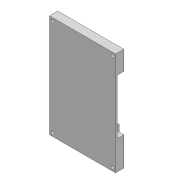
# Autodesk Inventor part: DE10-Nano
Saved by Autodesk Inventor 2018 (Build 220112000, 112)
## iProperties
Created: 2019-08-31
Part Number: DE10-Nano
Material: Generic
Document SubType Name: Modeling
Designer: Clevo
Density: 1 g/cm^3
Appearance: Default
Author: Clevo
Autodesk Inventor part; units mm, degrees
ref_plane "YZ Plane" through (0, 0, 0) normal (1, 0, 0) x (0, 1, 0)
ref_plane "XZ Plane" through (0, 0, 0) normal (0, 1, 0) x (-1, 0, 0)
ref_plane "XY Plane" through (0, 0, 0) normal (0, 0, 1) x (1, 0, 0)
sketch "Sketch1" plane through (0, 0, 0) normal (0, 1, 0) x (-1, 0, 0)
  line L0 (-34.295, -53.46) -> (34.295, -53.46)
  line L1 (34.295, -53.46) -> (34.295, 53.46)
  line L2 (34.295, 53.46) -> (-34.295, 53.46)
  line L3 (-34.295, 53.46) -> (-34.295, -53.46)
  line L4 (-34.295, -53.46) -> (34.295, 53.46) construction
  line L5 (34.295, -53.46) -> (-34.295, 53.46) construction
  point P0 (0, 0)
  dimension "d0" = 106.92
  dimension "d1" = 68.59
  constraints: 12 end point, 2 midpoint, 2 parallel, 1 horizontal, 1 perpendicular
  measures "d0" distance of L0.end L1.end
  measures "d1" distance of L1.end L2.end
extrude "Extrusion1" add sketch "Sketch1" along normal blind 1.6
sketch "Sketch2" plane through (0, 1.6, 0) normal (0, 1, 0) x (1, 0, 0)
  line L0 (-34.295, 53.46) -> (-34.295, -53.46) projected
  line L1 (34.295, -53.46) -> (34.295, 53.46) projected
  line L2 (-34.295, -53.46) -> (34.295, -53.46)
  line L3 (34.295, -53.46) -> (34.295, -33.46)
  line L4 (34.295, -33.46) -> (-34.295, -33.46)
  line L5 (-34.295, -33.46) -> (-34.295, -53.46)
  line L6 (34.295, 53.46) -> (-34.295, 53.46) projected
  line L7 (34.295, 53.46) -> (-34.295, 53.46)
  line L8 (-34.295, 53.46) -> (-34.295, 23.46)
  line L9 (-34.295, 23.46) -> (34.295, 23.46)
  line L10 (34.295, 23.46) -> (34.295, 53.46)
  point P0 (0, 0)
  dimension "d4" = 20
  dimension "d5" = 30
  constraints: 16 end point, 4 parallel, 2 horizontal, 2 perpendicular, 2 point on line
  measures "d4" distance between parallel lines of L2 L4
  measures "d5" distance between parallel lines of L6 L9
extrude "Extrusion2" add sketch "Sketch2" along normal blind 7 contours L6 L1 L9 L0 | L4 L1 L2 L0
sketch "Sketch3" plane through (0, 8.6, 0) normal (0, 1, 0) x (1, 0, 0)
  line L0 (34.295, 23.46) -> (-34.295, 23.46) projected
  line L1 (22.365, 53.46) -> (6.365, 53.46)
  line L2 (6.365, 53.46) -> (6.365, 23.46)
  line L3 (6.365, 23.46) -> (22.365, 23.46)
  line L4 (22.365, 23.46) -> (22.365, 53.46)
  line L5 (22.365, 53.46) -> (6.365, 23.46) construction
  line L6 (6.365, 53.46) -> (22.365, 23.46) construction
  line L7 (34.295, 53.46) -> (-34.295, 53.46) projected
  line L8 (34.295, 23.46) -> (34.295, 53.46) projected
  point P0 (0, 0)
  point P1 (14.365, 38.46)
  dimension "d8" = 19.93
  dimension "d9" = 16
  constraints: 12 end point, 2 midpoint, 2 parallel, 1 collinear, 1 horizontal, 1 perpendicular, 1 point on line
  measures "d8" distance from line of L8 point (14.365, 38.46)
  measures "d9" distance of L1.start L1.end
extrude "Extrusion3" add sketch "Sketch3" along normal blind 7 contours L0 L2 L1 L4
sketch "Sketch4" plane through (34.295, 0, -53.46) normal (0, 0, -1) x (-1, 0, 0)
  line L0 (13.93, 13.6) -> (25.93, 13.6)
  line L1 (25.93, 13.6) -> (25.93, 3.6)
  line L2 (25.93, 3.6) -> (13.93, 3.6)
  line L3 (13.93, 3.6) -> (13.93, 13.6)
  line L4 (11.93, 15.6) -> (27.93, 15.6) projected
  point P0 (34.295, 0)
  point P1 (25.93, 8.6)
  point P2 (27.93, 8.6)
  point P3 (19.93, 13.6)
  point P4 (19.93, 15.6)
  dimension "d12" = 12
  dimension "d13" = 10
  constraints: 8 end point, 3 midpoint, 2 parallel, 1 horizontal, 1 horizontal alignment, 1 perpendicular, 1 vertical alignment
  measures "d12" distance of L0.start L0.end
  measures "d13" distance of L0.end L1.end
extrude "Extrusion4" cut sketch "Sketch4" against normal blind 7
sketch "Sketch5" plane through (0, 8.6, 0) normal (0, 1, 0) x (1, 0, 0)
  line L0 (-31.115, -50.28) -> (31.115, -50.28)
  line L1 (31.115, -50.28) -> (31.115, 50.16)
  line L2 (31.115, 50.16) -> (-31.115, 50.16)
  line L3 (-31.115, 50.16) -> (-31.115, -50.28)
  line L4 (-34.295, -53.46) -> (34.295, -53.46) projected
  line L5 (34.295, -53.46) -> (34.295, -33.46) projected
  line L6 (-34.295, -33.46) -> (-34.295, -53.46) projected
  line L7 (6.365, 53.46) -> (-34.295, 53.46) projected
  point P0 (0, 0)
  dimension "d16" = 3.18
  dimension "d17" = 3.18
  dimension "d18" = 3.18
  dimension "d19" = 3.3
  constraints: 8 end point, 2 parallel, 1 horizontal, 1 perpendicular
  measures "d16" distance between parallel lines of L4 L0
  measures "d17" distance between parallel lines of L5 L1
  measures "d18" distance between parallel lines of L6 L3
  measures "d19" distance between parallel lines of L7 L2
hole "Hole1" at (-31.115, 8.6, 50.28) at (-31.115, 8.6, -50.16) at (31.115, 8.6, -50.16) at (31.115, 8.6, 50.28) direction (0, -1, 0) diameter 3.2 end through all clearance for "Flat Head Machine Screw" size "M3" standard "Ansi Metric M Profile"
sketch "Sketch6" plane through (0, 1.6, 0) normal (0, 1, 0) x (1, 0, 0)
  line L0 (-18, -12) -> (6, -12)
  line L1 (6, -12) -> (6, 12)
  line L2 (6, 12) -> (-18, 12)
  line L3 (-18, 12) -> (-18, -12)
  line L4 (-18, -12) -> (6, 12) construction
  line L5 (6, -12) -> (-18, 12) construction
  point P0 (0, 0)
  point P1 (-6, 0)
  point P2 (-6, 0)
  dimension "d27" = 24
  dimension "d28" = 24
  dimension "d29" = 6
  constraints: 12 end point, 3 midpoint, 2 parallel, 1 horizontal, 1 horizontal alignment, 1 perpendicular
  measures "d27" distance of L1.end L2.end
  measures "d28" distance of L2.end L0.start
  measures "d29" distance of point (0, 0) point (-6, 0)
extrude "Extrusion5" add sketch "Sketch6" along normal blind 3
sketch "Sketch7" plane through (0, 4.6, 0) normal (0, 1, 0) x (1, 0, 0)
  line L0 (-16.4012, 1.4056) -> (4.5001, 1.4056) construction
  line L1 (4.5001, 1.4056) -> (4.5001, -1.7684) construction
  line L2 (4.5001, -1.7684) -> (-16.4012, -1.7684) construction
  line L3 (-16.4012, -1.7684) -> (-16.4012, 1.4056) construction
  spline S0 degree 2 poles (-13.6891, -0.1826) (-13.6891, -0.6) (-14.0275, -1.2719) (-14.3116, -1.4596) knots 0 0 0 1 2 2 2
  spline S1 degree 2 poles (-14.3116, -1.4596) (-14.5437, -1.6053) (-15.0205, -1.7041) (-15.391, -1.7041) knots 0 0 0 1 2 2 2
  line L4 (-15.391, -1.7041) -> (-16.0924, -1.7041)
  line L5 (-16.0924, -1.7041) -> (-16.0924, 1.3439)
  line L6 (-16.0924, 1.3439) -> (-15.3984, 1.3439)
  spline S2 degree 2 poles (-15.3984, 1.3439) (-14.9686, 1.3439) (-14.4795, 1.2154) (-14.3066, 1.1018) knots 0 0 0 1 2 2 2
  spline S3 degree 2 poles (-14.3066, 1.1018) (-14.0127, 0.9067) (-13.6891, 0.262) (-13.6891, -0.1826) knots 0 0 0 1 2 2 2
  spline S4 degree 2 poles (-14.1115, -0.1777) (-14.1115, 0.1731) (-14.3437, 0.6695) (-14.5734, 0.8103) knots 0 0 0 1 2 2 2
  spline S5 degree 2 poles (-14.5734, 0.8103) (-14.7364, 0.9067) (-15.1044, 0.9931) (-15.3786, 0.9931) knots 0 0 0 1 2 2 2
  line L7 (-15.3786, 0.9931) -> (-15.6874, 0.9931)
  line L8 (-15.6874, 0.9931) -> (-15.6874, -1.3534)
  line L9 (-15.6874, -1.3534) -> (-15.3786, -1.3534)
  spline S6 degree 2 poles (-15.3786, -1.3534) (-15.1094, -1.3534) (-14.7018, -1.267) (-14.5363, -1.1509) knots 0 0 0 1 2 2 2
  spline S7 degree 2 poles (-14.5363, -1.1509) (-14.3239, -1.0076) (-14.1115, -0.5334) (-14.1115, -0.1777) knots 0 0 0 1 2 2 2
  line L10 (-13.2495, -1.7041) -> (-13.2495, 1.3439)
  line L11 (-13.2495, 1.3439) -> (-11.3426, 1.3439)
  line L12 (-11.3426, 1.3439) -> (-11.3426, 0.9832)
  line L13 (-11.3426, 0.9832) -> (-12.8444, 0.9832)
  line L14 (-12.8444, 0.9832) -> (-12.8444, 0.1484)
  line L15 (-12.8444, 0.1484) -> (-11.4439, 0.1484)
  line L16 (-11.4439, 0.1484) -> (-11.4439, -0.2123)
  line L17 (-11.4439, -0.2123) -> (-12.8444, -0.2123)
  line L18 (-12.8444, -0.2123) -> (-12.8444, -1.3435)
  line L19 (-12.8444, -1.3435) -> (-11.3426, -1.3435)
  line L20 (-11.3426, -1.3435) -> (-11.3426, -1.7041)
  line L21 (-11.3426, -1.7041) -> (-13.2495, -1.7041)
  line L22 (-9.2579, -1.7041) -> (-10.7449, -1.7041)
  line L23 (-10.7449, -1.7041) -> (-10.7449, -1.3929)
  line L24 (-10.7449, -1.3929) -> (-10.1916, -1.3929)
  line L25 (-10.1916, -1.3929) -> (-10.1916, 0.6498)
  line L26 (-10.1916, 0.6498) -> (-10.7449, 0.6498)
  line L27 (-10.7449, 0.6498) -> (-10.7449, 0.9289)
  spline S8 degree 2 poles (-10.7449, 0.9289) (-10.4312, 0.9289) (-10.1348, 1.1067) (-10.115, 1.3537) knots 0 0 0 1 2 2 2
  line L28 (-10.115, 1.3537) -> (-9.7988, 1.3537)
  line L29 (-9.7988, 1.3537) -> (-9.7988, -1.3929)
  line L30 (-9.7988, -1.3929) -> (-9.2579, -1.3929)
  line L31 (-9.2579, -1.3929) -> (-9.2579, -1.7041)
  spline S9 degree 2 poles (-6.8002, -0.1801) (-6.8002, -1.0002) (-7.277, -1.7684) (-7.7734, -1.7684) knots 0 0 0 1 2 2 2
  spline S10 degree 2 poles (-7.7734, -1.7684) (-8.2773, -1.7684) (-8.7491, -0.9854) (-8.7491, -0.1826) knots 0 0 0 1 2 2 2
  spline S11 degree 2 poles (-8.7491, -0.1826) (-8.7491, 0.6424) (-8.2724, 1.4056) (-7.7734, 1.4056) knots 0 0 0 1 2 2 2
  spline S12 degree 2 poles (-7.7734, 1.4056) (-7.272, 1.4056) (-6.8002, 0.6152) (-6.8002, -0.1801) knots 0 0 0 1 2 2 2
  spline S13 degree 2 poles (-7.3239, -1.1089) (-7.2646, -0.9582) (-7.2152, -0.4938) (-7.2152, -0.1801) knots 0 0 0 1 2 2 2
  spline S14 degree 2 poles (-7.2152, -0.1801) (-7.2152, 0.1335) (-7.2646, 0.5954) (-7.3264, 0.7511) knots 0 0 0 1 2 2 2
  spline S15 degree 2 poles (-7.3264, 0.7511) (-7.3881, 0.9067) (-7.603, 1.0672) (-7.7734, 1.0672) knots 0 0 0 1 2 2 2
  spline S16 degree 2 poles (-7.7734, 1.0672) (-7.9439, 1.0672) (-8.1637, 0.9067) (-8.2279, 0.7461) knots 0 0 0 1 2 2 2
  spline S17 degree 2 poles (-8.2279, 0.7461) (-8.2897, 0.5905) (-8.3341, 0.1163) (-8.3341, -0.1826) knots 0 0 0 1 2 2 2
  spline S18 degree 2 poles (-8.3341, -0.1826) (-8.3341, -0.5037) (-8.2946, -0.9335) (-8.2304, -1.1015) knots 0 0 0 1 2 2 2
  spline S19 degree 2 poles (-8.2304, -1.1015) (-8.1711, -1.2595) (-7.9513, -1.43) (-7.7734, -1.43) knots 0 0 0 1 2 2 2
  spline S20 degree 2 poles (-7.7734, -1.43) (-7.6055, -1.43) (-7.3856, -1.2694) (-7.3239, -1.1089) knots 0 0 0 1 2 2 2
  line L32 (-5.2935, -0.5556) -> (-6.447, -0.5556)
  line L33 (-6.447, -0.5556) -> (-6.447, -0.1851)
  line L34 (-6.447, -0.1851) -> (-5.2935, -0.1851)
  line L35 (-5.2935, -0.1851) -> (-5.2935, -0.5556)
  line L36 (-2.621, -1.7041) -> (-3.0755, -1.7041)
  line L37 (-3.0755, -1.7041) -> (-4.4241, 0.924)
  line L38 (-4.4241, 0.924) -> (-4.4241, -1.7041)
  line L39 (-4.4241, -1.7041) -> (-4.802, -1.7041)
  line L40 (-4.802, -1.7041) -> (-4.802, 1.3439)
  line L41 (-4.802, 1.3439) -> (-4.2265, 1.3439)
  line L42 (-4.2265, 1.3439) -> (-2.9989, -1.0693)
  line L43 (-2.9989, -1.0693) -> (-2.9989, 1.3439)
  line L44 (-2.9989, 1.3439) -> (-2.621, 1.3439)
  line L45 (-2.621, 1.3439) -> (-2.621, -1.7041)
  spline S21 degree 2 poles (-0.7586, -1.4621) (-0.8055, -1.4967) (-0.9636, -1.6202) (-1.0377, -1.6572) knots 0 0 0 1 2 2 2
  spline S22 degree 2 poles (-1.0377, -1.6572) (-1.139, -1.7116) (-1.3292, -1.7684) (-1.5021, -1.7684) knots 0 0 0 1 2 2 2
  spline S23 degree 2 poles (-1.5021, -1.7684) (-1.6429, -1.7684) (-1.8973, -1.6622) (-1.9936, -1.5658) knots 0 0 0 1 2 2 2
  spline S24 degree 2 poles (-1.9936, -1.5658) (-2.085, -1.472) (-2.1961, -1.1953) (-2.1961, -1.0422) knots 0 0 0 1 2 2 2
  spline S25 degree 2 poles (-2.1961, -1.0422) (-2.1961, -0.8051) (-1.9961, -0.4691) (-1.7787, -0.3728) knots 0 0 0 1 2 2 2
  spline S26 degree 2 poles (-1.7787, -0.3728) (-1.586, -0.2839) (-1.0624, -0.2172) (-0.7586, -0.1999) knots 0 0 0 1 2 2 2
  line L46 (-0.7586, -0.1999) -> (-0.7586, -0.1258)
  spline S27 degree 2 poles (-0.7586, -0.1258) (-0.7586, 0.0076) (-0.8401, 0.1731) (-0.9142, 0.22) knots 0 0 0 1 2 2 2
  spline S28 degree 2 poles (-0.9142, 0.22) (-0.9883, 0.2669) (-1.2007, 0.2966) (-1.3143, 0.2966) knots 0 0 0 1 2 2 2
  spline S29 degree 2 poles (-1.3143, 0.2966) (-1.4477, 0.2966) (-1.8083, 0.2175) (-1.9887, 0.141) knots 0 0 0 1 2 2 2
  line L47 (-1.9887, 0.141) -> (-2.0109, 0.141)
  line L48 (-2.0109, 0.141) -> (-2.0109, 0.5337)
  spline S30 degree 2 poles (-2.0109, 0.5337) (-1.9047, 0.5633) (-1.507, 0.6374) (-1.3119, 0.6374) knots 0 0 0 1 2 2 2
  spline S31 degree 2 poles (-1.3119, 0.6374) (-1.0747, 0.6374) (-0.7512, 0.5633) (-0.6227, 0.467) knots 0 0 0 1 2 2 2
  spline S32 degree 2 poles (-0.6227, 0.467) (-0.4968, 0.3731) (-0.3733, 0.0743) (-0.3733, -0.1406) knots 0 0 0 1 2 2 2
  line L49 (-0.3733, -0.1406) -> (-0.3733, -1.7041)
  line L50 (-0.3733, -1.7041) -> (-0.7586, -1.7041)
  line L51 (-0.7586, -1.7041) -> (-0.7586, -1.4621)
  line L52 (-0.7586, -1.141) -> (-0.7586, -0.5062)
  spline S33 degree 2 poles (-0.7586, -0.5062) (-0.8969, -0.5185) (-1.3143, -0.5605) (-1.4453, -0.6) knots 0 0 0 1 2 2 2
  spline S34 degree 2 poles (-1.4453, -0.6) (-1.5984, -0.647) (-1.7985, -0.8421) (-1.7985, -1.015) knots 0 0 0 1 2 2 2
  spline S35 degree 2 poles (-1.7985, -1.015) (-1.7985, -1.2126) (-1.5762, -1.4127) (-1.3637, -1.4127) knots 0 0 0 1 2 2 2
  spline S36 degree 2 poles (-1.3637, -1.4127) (-1.1834, -1.4127) (-0.887, -1.2571) (-0.7586, -1.141) knots 0 0 0 1 2 2 2
  line L53 (1.9634, -1.7041) -> (1.578, -1.7041)
  line L54 (1.578, -1.7041) -> (1.578, -0.4)
  spline S37 degree 2 poles (1.578, -0.4) (1.578, -0.2419) (1.5484, 0.0298) (1.5039, 0.1113) knots 0 0 0 1 2 2 2
  spline S38 degree 2 poles (1.5039, 0.1113) (1.457, 0.1978) (1.2891, 0.2817) (1.1458, 0.2817) knots 0 0 0 1 2 2 2
  spline S39 degree 2 poles (1.1458, 0.2817) (1.0025, 0.2817) (0.6987, 0.1286) (0.553, 0.0051) knots 0 0 0 1 2 2 2
  line L55 (0.553, 0.0051) -> (0.553, -1.7041)
  line L56 (0.553, -1.7041) -> (0.1677, -1.7041)
  line L57 (0.1677, -1.7041) -> (0.1677, 0.5831)
  line L58 (0.1677, 0.5831) -> (0.553, 0.5831)
  line L59 (0.553, 0.5831) -> (0.553, 0.3287)
  spline S40 degree 2 poles (0.553, 0.3287) (0.7259, 0.4843) (1.0593, 0.6473) (1.2471, 0.6473) knots 0 0 0 1 2 2 2
  spline S41 degree 2 poles (1.2471, 0.6473) (1.583, 0.6473) (1.9634, 0.2027) (1.9634, -0.2197) knots 0 0 0 1 2 2 2
  line L60 (1.9634, -0.2197) -> (1.9634, -1.7041)
  spline S42 degree 2 poles (4.384, -0.5605) (4.384, -1.1385) (3.8282, -1.7684) (3.3639, -1.7684) knots 0 0 0 1 2 2 2
  spline S43 degree 2 poles (3.3639, -1.7684) (2.8872, -1.7684) (2.3413, -1.1188) (2.3413, -0.5605) knots 0 0 0 1 2 2 2
  spline S44 degree 2 poles (2.3413, -0.5605) (2.3413, 0.0125) (2.9044, 0.6473) (3.3639, 0.6473) knots 0 0 0 1 2 2 2
  spline S45 degree 2 poles (3.3639, 0.6473) (3.8282, 0.6473) (4.384, 0.015) (4.384, -0.5605) knots 0 0 0 1 2 2 2
  spline S46 degree 2 poles (3.9863, -0.5605) (3.9863, -0.1159) (3.6627, 0.3163) (3.3639, 0.3163) knots 0 0 0 1 2 2 2
  spline S47 degree 2 poles (3.3639, 0.3163) (3.065, 0.3163) (2.739, -0.1159) (2.739, -0.5605) knots 0 0 0 1 2 2 2
  spline S48 degree 2 poles (2.739, -0.5605) (2.739, -0.9928) (3.065, -1.4374) (3.3639, -1.4374) knots 0 0 0 1 2 2 2
  spline S49 degree 2 poles (3.3639, -1.4374) (3.6603, -1.4374) (3.9863, -1.0002) (3.9863, -0.5605) knots 0 0 0 1 2 2 2
  point P0 (0, 0)
  constraints: 2 other
extrude "Extrusion6" add sketch "Sketch7" along normal blind 1
equation "\"d28\" = d27"
body "Solid1"
